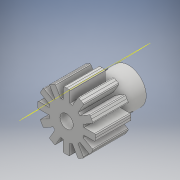
# Autodesk Inventor part: Część1
Saved by Autodesk Inventor 2017 (Build 210142000, 142)
## iProperties
Created: 2017-01-08
Part Number: Część1
Material: Ogólny
Document SubType Name: Modeling
Designer: Cwaluch
Density: 1 g/cm^3
Appearance: Domyślna
Author: Cwaluch
Autodesk Inventor part; units mm, degrees
ref_plane "YZ Plane" through (0, 0, 0) normal (1, 0, 0) x (0, 1, 0)
ref_plane "XZ Plane" through (0, 0, 0) normal (0, 1, 0) x (-1, 0, 0)
ref_plane "XY Plane" through (0, 0, 0) normal (0, 0, 1) x (1, 0, 0)
sketch "Szkic1" plane through (0, 0, 0) normal (0, 1, 0) x (-1, 0, 0)
  circle A0 centre (0, 0) radius 4
  dimension "d0" = 8
  constraints: 1 centre point, 1 coincident
  measures "d0" diameter of A0
extrude "Wyciągnięcie proste1" add sketch "Szkic1" along normal blind 8
sketch "Szkic3" plane through (0, 8, 0) normal (0, 1, 0) x (1, 0, 0)
  circle A0 centre (0, 0) radius 4 projected
  line L0 (-6.5052, -0.0059) -> (-6.5011, 0.744)
  line L1 (-6.5052, -0.0059) -> (-6.5052, -0.7559)
  line L2 (-6.5052, -0.7559) -> (-3.9279, -0.7559)
  line L3 (-6.5011, 0.744) -> (-3.9302, 0.744)
  line L4 (-6.5011, 0.744) -> (-3.9302, 0.744) construction
  dimension "d5" = 0.75
  dimension "d6" = 0.75
  dimension "d7" = 0
  dimension "d8" = 2.5709
  dimension "d9" = 2.5773
  constraints: 10 end point, 2 point on circle, 1 collinear, 1 horizontal, 1 parallel, 1 vertical
  measures "d5" distance of L0.start L0.end
  measures "d6" distance of L0.start L1.end
  measures "d7" distance between parallel lines of L3 L4
  measures "d8" distance of L0.end L3.end
  measures "d9" distance of L1.end L2.end
extrude "Wyciągnięcie proste2" add sketch "Szkic3" against normal blind 8 contours A0 L2 L1 L0 L3
pattern_circular "Szyk kołowy1" count 12 over 360 about axis through (0, 0, 0) along (0, 1, 0) of "Wyciągnięcie proste2"
fillet "Zaokrąglenie1" radius 0.2 24 edges at (-5.2581, 4, -3.8949) (-6.0117, 4, -2.598) (-2.6062, 4, -6.0022) (-3.9073, 4, -5.2557) (-0.7559, 4, -6.5052) (0.744, 4, -6.5011) (2.598, 4, -6.0117) (3.8949, 4, -5.2581) (5.2557, 4, -3.9073) (6.0022, 4, -2.6062) (6.5052, 4, -0.7559) (6.5011, 4, 0.744) (6.0117, 4, 2.598) (5.2581, 4, 3.8949) (3.9073, 4, 5.2557) (2.6062, 4, 6.0022) (0.7559, 4, 6.5052) (-0.744, 4, 6.5011) (-2.598, 4, 6.0117) (-3.8949, 4, 5.2581) (-5.2557, 4, 3.9073) (-6.0022, 4, 2.6062) (-6.5052, 4, 0.7559) (-6.5011, 4, -0.744)
sketch "Szkic4" plane through (0, 8, 0) normal (0, 1, 0) x (1, 0, 0)
  circle A0 centre (0, 0) radius 4
  dimension "d16" = 8
  constraints: 1 centre point, 1 coincident
  measures "d16" diameter of A0
extrude "Wyciągnięcie proste3" add sketch "Szkic4" along normal blind 6
ref_plane "Płaszczyzna konstrukcyjna1" through (-6.3022, 8, -0.744) normal (-0.7169946, 0, 0.6970787) x (0, -1, 0)
sketch "Szkic5" plane through (-6.3022, 8, -0.744) normal (-0.7169946, 0, 0.6970787) x (0, -1, 0)
  circle A0 centre (-3, 4.9266) radius 1
  point P0 (8, 4.9266)
  dimension "d19" = 2
  constraints: 1 centre point
  measures "d19" diameter of A0
extrude "Wyciągnięcie proste4" cut sketch "Szkic5" against normal through all
sketch "Szkic6" plane through (0, 14, 0) normal (0, 1, 0) x (1, 0, 0)
  circle A0 centre (0, 0) radius 1.5
  dimension "d22" = 3
  constraints: 1 centre point, 1 coincident
  measures "d22" diameter of A0
extrude "Wyciągnięcie proste5" cut sketch "Szkic6" against normal through all
